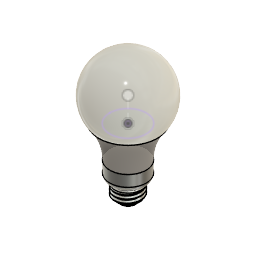
Light_bulb (Autodesk Fusion 360 design; units mm, degrees)
part number: 2026-02-19-17-51-17-661
Autodesk Fusion 360 part; units mm, degrees
cylinder "CylinderPrimitive1" add diameter 30 height 40 placed x (1, 0, 0) y (0, 1, 0) z (0, 0, 1) at (0, 0, 0) makes body 1
sketch "Sketch2" plane through (0, 0, 0) normal (0, 1, 0) x (1, 0, 0)
  circle A0 through (-15, -40, 0) (7.5, -40, 12.9904) (7.5, -40, -12.9904)
  line L0 (0, -40) -> (0, -60) construction
  dimension "d3" = 20
  constraint vertical L0
  measures "d3" distance of L0.start L0.end
sphere "SpherePrimitive1" add diameter 61 placed x (1, 0, 0) y (0, 0, -1) z (0, 1, 0) at (0, 0, 60) bodies 1
fillet "Fillet1" radius 45 1 edges at (-13.9849, 5.4242, 33.4435) on bodies 1
fillet "Fillet2" radius 5 1 edges at (-13.9849, 5.4242, 0) on bodies 1
cylinder "CylinderPrimitive2" add diameter 22 height 15 placed x (0, 1, 0) y (1, 0, 0) z (0, 0, -1) at (0, 0, 0) separate body makes body 2
thread "Thread1" "ANSI Metric M Profile 22.0 M22x3 M22x3 6g" major diameter 21.7645 minor diameter 18.3374 pitch 3 angle 60 modelled right hand crest width 0.4298 on face at (-1.0952, 10.9453, -5) from (0, 0, -2) to (0, 0, -12) crest through (0, 10.8823, 0.75) on bodies 2
chamfer "Chamfer1" distance 5 angle 45 1 edges at (-3.9352, -10.1458, -15) on bodies 2
fillet "Fillet3" radius 2 1 edges at (2.1271, -5.4842, -15) on bodies 2
cylinder "CylinderPrimitive3" add diameter 10.108 height 2 placed x (0, 1, 0) y (1, 0, 0) z (0, 0, -1) at (0, 0, -15) bodies 2
chamfer "Chamfer2" distance 2 angle 45 1 edges at (-1.8276, -4.712, -17) on bodies 2
